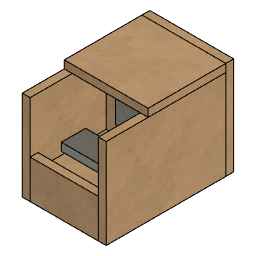
ERK-1 (Autodesk Fusion 360 design; units mm, degrees)
Autodesk Fusion 360 part; units mm, degrees
ref_plane "WorkPlane1" through (0, 0, 60) normal (0, 0, 1) x (1, 0, 0) in component "Base"
sketch "Sketch1" plane through (0, 0, 60) normal (0, 0, 1) x (1, 0, 0) in component "Base"
  line L0 (122, -122) -> (-122, -122)
  line L1 (-122, -122) -> (-122, 122)
  line L2 (-122, 122) -> (122, 122)
  line L3 (122, 122) -> (122, -122)
  line L4 (122, -122) -> (-122, 122) construction
  line L5 (-122, -122) -> (122, 122) construction
  dimension "d8" = 244
  dimension "d9" = 244
  constraint horizontal L0
  constraint perpendicular L0 L1
  constraint parallel L0 L2
  constraint parallel L1 L3
  constraint coincident L4 origin
  constraint coincident L5 origin
  measures "d8" distance of L1.end L2.end
  measures "d9" distance of L0.end L1.end
extrude "Extrude1" add sketch "Sketch1" along normal blind 28 makes body 1 in component "Base"
ref_plane "WorkPlane1" through (0, -122, 0) normal (0, 1, 0) x (0, 0, 1) in component "Front"
sketch "Sketch1 (2)" plane through (0, -122, 0) normal (0, 1, 0) x (1, 0, 0) in component "Front"
  line L0 (122, 0) -> (-122, 0)
  line L1 (-122, 0) -> (-122, -138)
  line L2 (-122, -138) -> (122, -138)
  line L3 (122, -138) -> (122, 0)
  line L4 (122, 0) -> (-122, -138) construction
  line L5 (-122, 0) -> (122, -138) construction
  point P0 (0, -69)
  dimension "d15" = 244
  dimension "d16" = 138
  constraint horizontal L0
  constraint perpendicular L0 L1
  constraint parallel L0 L2
  constraint parallel L1 L3
  constraint coincident L4 P0
  constraint coincident L5 P0
  constraint midpoint L0 origin
  measures "d15" distance of L1.end L2.end
  measures "d16" distance of L0.end L1.end
extrude "Extrude1'" add sketch "Sketch1 (2)" against normal blind 28 separate body makes body 2 in component "Front"
ref_plane "WorkPlane1" through (0, 122, 0) normal (0, 1, 0) x (0, 0, 1) in component "Rear"
sketch "Sketch1 (3)" plane through (0, 122, 0) normal (0, 1, 0) x (1, 0, 0) in component "Rear"
  line L0 (-122, -322) -> (122, -322)
  line L1 (122, -322) -> (122, 0)
  line L2 (122, 0) -> (-122, 0)
  line L3 (-122, 0) -> (-122, -322)
  line L4 (-122, -322) -> (122, 0) construction
  line L5 (122, -322) -> (-122, 0) construction
  point P0 (0, -161)
  dimension "d21" = 244
  dimension "d22" = 322
  constraint horizontal L0
  constraint perpendicular L0 L1
  constraint parallel L0 L2
  constraint parallel L1 L3
  constraint coincident L4 P0
  constraint coincident L5 P0
  constraint midpoint L2 origin
  measures "d21" distance of L1.end L2.end
  measures "d22" distance of L0.end L1.end
extrude "Extrude1''" add sketch "Sketch1 (3)" along normal blind 28 separate body makes body 3 in component "Rear"
ref_plane "WorkPlane1" through (-122, 0, 0) normal (1, 0, 0) x (0, 1, 0) in component "Side"
sketch "Sketch1 (4)" plane through (-122, 0, 0) normal (1, 0, 0) x (0, 1, 0) in component "Side"
  line L0 (-150, 0) -> (278, 0)
  line L1 (278, 0) -> (278, 322)
  line L2 (278, 322) -> (-150, 322)
  line L3 (-150, 322) -> (-150, 0)
  line L4 (-150, 0) -> (278, 322) construction
  line L5 (278, 0) -> (-150, 322) construction
  point P0 (64, 161)
  dimension "d26" = 428
  dimension "d27" = 322
  dimension "d32" = 150
  constraint horizontal L0
  constraint perpendicular L0 L1
  constraint parallel L0 L2
  constraint parallel L1 L3
  constraint coincident L4 P0
  constraint coincident L5 P0
  constraint coincident origin L0
  measures "d26" distance of L1.end L2.end
  measures "d27" distance of L0.end L1.end
  measures "d32" distance of origin L3
extrude "Extrude1'''" add sketch "Sketch1 (4)" against normal blind 28 separate body makes body 4 in component "Side"
ref_plane "WorkPlane1" through (0, 0, 322) normal (0, 0, 1) x (1, 0, 0) in component "Top"
sketch "Sketch1 (5)" plane through (0, 0, 322) normal (0, 0, 1) x (1, 0, 0) in component "Top"
  line L0 (-150, 278) -> (150, 278)
  line L1 (150, 278) -> (150, 0)
  line L2 (150, 0) -> (-150, 0)
  line L3 (-150, 0) -> (-150, 278)
  dimension "d36" = 300
  dimension "d38" = 278
  constraint horizontal L0
  constraint vertical L1
  constraint horizontal L2
  constraint vertical L3
  constraint midpoint L2 origin
  measures "d36" distance of L0.start L0.end
  measures "d38" distance of L0.end L1.end
extrude "Extrude1''''" add sketch "Sketch1 (5)" along normal blind 28 separate body makes body 5 in component "Top"
ref_plane "WorkPlane1" through (0, 278, 0) normal (0, 1, 0) x (0, 0, 1) in component "RearCap"
sketch "Sketch1 (6)" plane through (0, 278, 0) normal (0, 1, 0) x (1, 0, 0) in component "RearCap"
  line L0 (150, -350) -> (-150, -350)
  line L1 (-150, -350) -> (-150, 0)
  line L2 (-150, 0) -> (150, 0)
  line L3 (150, 0) -> (150, -350)
  dimension "d42" = 300
  dimension "d43" = 350
  constraint horizontal L0
  constraint vertical L1
  constraint horizontal L2
  constraint vertical L3
  constraint midpoint L2 origin
  measures "d42" distance of L0.start L0.end
  measures "d43" distance of L0.end L1.end
extrude "Extrude1'''''" add sketch "Sketch1 (6)" along normal blind 28 separate body makes body 6 in component "RearCap"
ref_plane "WorkPlane1" through (0, 0, 138) normal (0, 0, 1) x (1, 0, 0) in component "SpoilBoard"
sketch "Sketch1 (7)" plane through (0, 0, 138) normal (0, 0, 1) x (1, 0, 0) in component "SpoilBoard"
  line L0 (112, -43.4103) -> (-112, -43.4103)
  line L1 (-112, -43.4103) -> (-112, 43.4103)
  line L2 (-112, 43.4103) -> (112, 43.4103)
  line L3 (112, 43.4103) -> (112, -43.4103)
  line L4 (112, -43.4103) -> (-112, 43.4103) construction
  line L5 (-112, -43.4103) -> (112, 43.4103) construction
  dimension "d49" = 224
  dimension "d50" = 86.8207
  constraint horizontal L0
  constraint perpendicular L0 L1
  constraint parallel L0 L2
  constraint parallel L1 L3
  constraint coincident L4 origin
  constraint coincident L5 origin
  measures "d49" distance of L1.end L2.end
  measures "d50" distance of L0.end L1.end
extrude "Extrude1''''''" add sketch "Sketch1 (7)" against normal blind 28 separate body makes body 7 in component "SpoilBoard"
ref_plane "WorkPlane1" through (0, 122, 0) normal (0, 1, 0) x (0, 0, 1) in component "X-Carriage"
ref_plane "WorkPlane2" through (0, 102, 0) normal (0, 1, 0) x (0, 0, 1) in component "X-Carriage"
sketch "Sketch1 (8)" plane through (0, 102, 0) normal (0, 1, 0) x (1, 0, 0) in component "X-Carriage"
  line L0 (-45, -318) -> (45, -318)
  line L1 (45, -318) -> (45, -218)
  line L2 (45, -218) -> (-45, -218)
  line L3 (-45, -218) -> (-45, -318)
  point P0 (0, -218)
  dimension "d64" = 90
  dimension "d65" = 100
  dimension "d66" = 218
  constraint horizontal L0
  constraint vertical L1
  constraint horizontal L2
  constraint vertical L3
  constraint midpoint L2 P0
  constraint vertical origin P0
  measures "d64" distance of L0.start L0.end
  measures "d65" distance of L0.end L1.end
  measures "d66" distance of origin L2
extrude "Extrude1'''''''" add sketch "Sketch1 (8)" against normal blind 28 separate body makes body 8 in component "X-Carriage"
component "Base" placed x (1, 0, 0) y (0, 1, 0) z (0, 0, 1) at (0, 0, 0)
component "Front" placed x (1, 0, 0) y (0, 1, 0) z (0, 0, 1) at (0, 0, 0)
component "Rear" placed x (1, 0, 0) y (0, 1, 0) z (0, 0, 1) at (0, 0, 0)
component "Side" placed x (1, 0, 0) y (0, 1, 0) z (0, 0, 1) at (0, 0, 0)
component "Top" placed x (1, 0, 0) y (0, 1, 0) z (0, 0, 1) at (0, 0, 0)
component "RearCap" placed x (1, 0, 0) y (0, 1, 0) z (0, 0, 1) at (0, 0, 0)
component "SpoilBoard" placed x (1, 0, 0) y (0, 1, 0) z (0, 0, 1) at (0, 63.3138, 0)
component "X-Carriage" placed x (1, 0, 0) y (0, 1, 0) z (0, 0, 1) at (0, 0, 0)
component "Side" placed x (1, 0, 0) y (0, 1, 0) z (0, 0, 1) at (272, 0, 0)
equation "frameThickness = 28 mm"
equation "outsideWidth = baseWidth + frameThickness * 2"
equation "outsideLength = baseLength + rearCavityLength + frameThickness * 3"
equation "bottomCavityHeight = 60 mm"
equation "baseWidth = 244 mm"
equation "baseLength = 244 mm"
equation "d7 = bottomCavityHeight"
equation "d8 = baseWidth"
equation "d9 = baseLength"
equation "d10 = frameThickness"
equation "frontLipHeight = bottomCavityHeight + frameThickness + baseBoxHeight"
equation "baseBoxHeight = 50 mm"
equation "d14 = -baseLength / 2"
equation "d15 = baseWidth"
equation "d16 = frontLipHeight"
equation "d17 = -frameThickness"
equation "d19 = baseLength / 2"
equation "outsideHeight = 350 mm"
equation "d21 = baseWidth"
equation "d22 = rearPanelHeight"
equation "d23 = frameThickness"
equation "d25 = -baseWidth / 2"
equation "d26 = outsideLength"
equation "d27 = sidePanelHeight"
equation "d28 = -frameThickness"
equation "rearCavityLength = 100 mm"
equation "sidePanelLength = outsideLength - frameThickness"
equation "d32 = baseLength / 2 + frameThickness"
equation "sidePanelHeight = outsideHeight - frameThickness"
equation "rearPanelHeight = sidePanelHeight"
equation "d35 = outsideHeight - frameThickness"
equation "d36 = outsideWidth"
equation "topPanelLength = outsideLength - baseLength / 2 - frameThickness"
equation "d38 = topPanelLength"
equation "d39 = frameThickness"
equation "d41 = outsideLength - baseLength / 2 - frameThickness"
equation "d42 = outsideWidth"
equation "d43 = outsideHeight"
equation "d44 = frameThickness"
equation "d46 = frontLipHeight"
equation "spoilBoardWidth = baseWidth - 20 mm"
equation "spoilBoardLength = baseLength / 2 - 20 mm"
equation "d49 = spoilBoardWidth"
equation "d51 = -frameThickness"
equation "d58 = baseLength - spoilBoardLength - 10 mm"
equation "d59 = baseLength / 2"
equation "xCarriageWidth = 90 mm"
equation "xCarriageHeight = 100 mm"
equation "xCarriageElevation = frontLipHeight + 80 mm"
equation "d64 = xCarriageWidth"
equation "d65 = xCarriageHeight"
equation "d66 = xCarriageElevation"
equation "d67 = -frameThickness"
